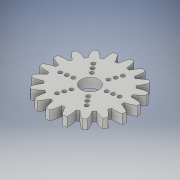
# Autodesk Inventor part: 000.303 - Шестерня привода
Saved by Autodesk Inventor 2019 (Build 230136000, 136)
## iProperties
Created: 2020-02-27
Part Number: 000.303 - Шестерня привода
Material: Типовые
Document SubType Name: Modeling
Designer: Петров Иван
Density: 1 g/cm^3
Appearance: По умолчанию
Author: Петров Иван
Autodesk Inventor part; units mm, degrees
ref_plane "YZ Plane" through (0, 0, 0) normal (1, 0, 0) x (0, 1, 0)
ref_plane "XZ Plane" through (0, 0, 0) normal (0, 1, 0) x (-1, 0, 0)
ref_plane "XY Plane" through (0, 0, 0) normal (0, 0, 1) x (1, 0, 0)
sketch "Эскиз1" plane through (0, 0, 0) normal (0, 1, 0) x (-1, 0, 0)
  arc A0 (-8.6049, 20.7741) -> (-8.0517, 15.4673) centre (8.9595, 19.9228) ccw
  arc A1 (-8.0517, 15.4673) -> (-9.3692, 14.7066) centre (0, 0) ccw
  arc A2 (-9.3692, 14.7066) -> (-13.6885, 17.8391) centre (-21.7334, 2.2022) ccw
  arc A3 (-13.6885, 17.8391) -> (-15.1912, 16.5782) centre (0, 0) ccw
  arc A4 (-15.1912, 16.5782) -> (-12.8563, 11.7806) centre (1.6052, 21.7856) ccw
  arc A5 (-12.8563, 11.7806) -> (-13.8341, 10.6153) centre (0, 0) ccw
  arc A6 (-13.8341, 10.6153) -> (-18.9643, 12.0816) centre (-21.1759, -5.3638) ccw
  arc A7 (-18.9643, 12.0816) -> (-19.9451, 10.3828) centre (0, 0) ccw
  arc A8 (-19.9451, 10.3828) -> (-16.1101, 6.673) centre (-5.9427, 21.0208) ccw
  arc A9 (-16.1101, 6.673) -> (-16.6304, 5.2436) centre (0, 0) ccw
  arc A10 (-16.6304, 5.2436) -> (-21.9528, 4.8668) centre (-18.0643, -12.2829) ccw
  arc A11 (-21.9528, 4.8668) -> (-22.2934, 2.935) centre (0, 0) ccw
  arc A12 (-22.2934, 2.935) -> (-17.4209, 0.7606) centre (-12.7739, 17.7205) ccw
  arc A13 (-17.4209, 0.7606) -> (-17.4209, -0.7606) centre (0, 0) ccw
  arc A14 (-17.4209, -0.7606) -> (-22.2934, -2.935) centre (-12.7739, -17.7205) ccw
  arc A15 (-22.2934, -2.935) -> (-21.9528, -4.8668) centre (0, 0) ccw
  arc A16 (-21.9528, -4.8668) -> (-16.6304, -5.2436) centre (-18.0643, 12.2829) ccw
  arc A17 (-16.6304, -5.2436) -> (-16.1101, -6.673) centre (0, 0) ccw
  arc A18 (-16.1101, -6.673) -> (-19.9451, -10.3828) centre (-5.9427, -21.0208) ccw
  arc A19 (-19.9451, -10.3828) -> (-18.9643, -12.0816) centre (0, 0) ccw
  arc A20 (-18.9643, -12.0816) -> (-13.8341, -10.6153) centre (-21.1759, 5.3638) ccw
  arc A21 (-13.8341, -10.6153) -> (-12.8563, -11.7806) centre (0, 0) ccw
  arc A22 (-12.8563, -11.7806) -> (-15.1912, -16.5782) centre (1.6052, -21.7856) ccw
  arc A23 (-15.1912, -16.5782) -> (-13.6885, -17.8391) centre (0, 0) ccw
  arc A24 (-13.6885, -17.8391) -> (-9.3692, -14.7066) centre (-21.7334, -2.2022) ccw
  arc A25 (-9.3692, -14.7066) -> (-8.0517, -15.4673) centre (0, 0) ccw
  arc A26 (-8.0517, -15.4673) -> (-8.6049, -20.7741) centre (8.9595, -19.9228) ccw
  arc A27 (-8.6049, -20.7741) -> (-6.7616, -21.445) centre (0, 0) ccw
  arc A28 (-6.7616, -21.445) -> (-3.7742, -17.0242) centre (-19.6695, -9.5027) ccw
  arc A29 (-3.7742, -17.0242) -> (-2.2761, -17.2883) centre (0, 0) ccw
  arc A30 (-2.2761, -17.2883) -> (-0.9808, -22.4644) centre (15.2332, -15.6569) ccw
  arc A31 (-0.9808, -22.4644) -> (0.9808, -22.4644) centre (0, 0) ccw
  arc A32 (0.9808, -22.4644) -> (2.2761, -17.2883) centre (-15.2332, -15.6569) ccw
  arc A33 (2.2761, -17.2883) -> (3.7742, -17.0242) centre (0, 0) ccw
  arc A34 (3.7742, -17.0242) -> (6.7616, -21.445) centre (19.6695, -9.5027) ccw
  arc A35 (6.7616, -21.445) -> (8.6049, -20.7741) centre (0, 0) ccw
  arc A36 (8.6049, -20.7741) -> (8.0517, -15.4673) centre (-8.9595, -19.9228) ccw
  arc A37 (8.0517, -15.4673) -> (9.3692, -14.7066) centre (0, 0) ccw
  arc A38 (9.3692, -14.7066) -> (13.6885, -17.8391) centre (21.7334, -2.2022) ccw
  arc A39 (13.6885, -17.8391) -> (15.1912, -16.5782) centre (0, 0) ccw
  arc A40 (15.1912, -16.5782) -> (12.8563, -11.7806) centre (-1.6052, -21.7856) ccw
  arc A41 (12.8563, -11.7806) -> (13.8341, -10.6153) centre (0, 0) ccw
  arc A42 (13.8341, -10.6153) -> (18.9643, -12.0816) centre (21.1759, 5.3638) ccw
  arc A43 (18.9643, -12.0816) -> (19.9451, -10.3828) centre (0, 0) ccw
  arc A44 (19.9451, -10.3828) -> (16.1101, -6.673) centre (5.9427, -21.0208) ccw
  arc A45 (16.1101, -6.673) -> (16.6304, -5.2436) centre (0, 0) ccw
  arc A46 (16.6304, -5.2436) -> (21.9528, -4.8668) centre (18.0643, 12.2829) ccw
  arc A47 (21.9528, -4.8668) -> (22.2934, -2.935) centre (0, 0) ccw
  arc A48 (22.2934, -2.935) -> (17.4209, -0.7606) centre (12.7739, -17.7205) ccw
  arc A49 (17.4209, -0.7606) -> (17.4209, 0.7606) centre (0, 0) ccw
  arc A50 (17.4209, 0.7606) -> (22.2934, 2.935) centre (12.7739, 17.7205) ccw
  arc A51 (22.2934, 2.935) -> (21.9528, 4.8668) centre (0, 0) ccw
  arc A52 (21.9528, 4.8668) -> (16.6304, 5.2436) centre (18.0643, -12.2829) ccw
  arc A53 (16.6304, 5.2436) -> (16.1101, 6.673) centre (0, 0) ccw
  arc A54 (16.1101, 6.673) -> (19.9451, 10.3828) centre (5.9427, 21.0208) ccw
  arc A55 (19.9451, 10.3828) -> (18.9643, 12.0816) centre (0, 0) ccw
  arc A56 (18.9643, 12.0816) -> (13.8341, 10.6153) centre (21.1759, -5.3638) ccw
  arc A57 (13.8341, 10.6153) -> (12.8563, 11.7806) centre (0, 0) ccw
  arc A58 (12.8563, 11.7806) -> (15.1912, 16.5782) centre (-1.6052, 21.7856) ccw
  arc A59 (15.1912, 16.5782) -> (13.6885, 17.8391) centre (0, 0) ccw
  arc A60 (13.6885, 17.8391) -> (9.3692, 14.7066) centre (21.7334, 2.2022) ccw
  arc A61 (9.3692, 14.7066) -> (8.0517, 15.4673) centre (0, 0) ccw
  arc A62 (8.0517, 15.4673) -> (8.6049, 20.7741) centre (-8.9595, 19.9228) ccw
  arc A63 (8.6049, 20.7741) -> (6.7616, 21.445) centre (0, 0) ccw
  arc A64 (6.7616, 21.445) -> (3.7742, 17.0242) centre (19.6695, 9.5027) ccw
  arc A65 (3.7742, 17.0242) -> (2.2761, 17.2883) centre (0, 0) ccw
  arc A66 (2.2761, 17.2883) -> (0.9808, 22.4644) centre (-15.2332, 15.6569) ccw
  arc A67 (0.9808, 22.4644) -> (-0.9808, 22.4644) centre (0, 0) ccw
  arc A68 (-0.9808, 22.4644) -> (-2.2761, 17.2883) centre (15.2332, 15.6569) ccw
  arc A69 (-2.2761, 17.2883) -> (-3.7742, 17.0242) centre (0, 0) ccw
  arc A70 (-3.7742, 17.0242) -> (-6.7616, 21.445) centre (-19.6695, 9.5027) ccw
  arc A71 (-6.7616, 21.445) -> (-8.6049, 20.7741) centre (0, 0) ccw
  constraints: 144 point on circle, 72 centre point
extrude "Выдавливание1" add sketch "Эскиз1" along normal blind 5
sketch "Эскиз2" plane through (0, 5, 0) normal (0, 1, 0) x (1, 0, 0)
  arc A0 (14.2029, 0.3107) -> (13.9664, 4.3996) centre (13.4768, 2.32) ccw
  line L0 (13.9664, 4.3996) -> (5.393, 4.3996)
  line L1 (5.393, 4.3996) -> (6.8323, 12.4554)
  arc A1 (6.8323, 12.4554) -> (3.173, 14.2951) centre (4.7292, 12.8312) ccw
  line L2 (3.173, 14.2951) -> (-1.1137, 6.8702)
  line L3 (-1.1137, 6.8702) -> (-7.3706, 12.1447)
  arc A2 (-7.3706, 12.1447) -> (-10.7934, 9.8955) centre (-8.7476, 10.5112) ccw
  line L4 (-10.7934, 9.8955) -> (-6.5067, 2.4706)
  line L5 (-6.5067, 2.4706) -> (-14.2029, -0.3107)
  arc A3 (-14.2029, -0.3107) -> (-13.9664, -4.3996) centre (-13.4768, -2.32) ccw
  line L6 (-13.9664, -4.3996) -> (-5.393, -4.3996)
  line L7 (-5.393, -4.3996) -> (-6.8323, -12.4554)
  arc A4 (-6.8323, -12.4554) -> (-3.173, -14.2951) centre (-4.7292, -12.8312) ccw
  line L8 (-3.173, -14.2951) -> (1.1137, -6.8702)
  line L9 (1.1137, -6.8702) -> (7.3706, -12.1447)
  arc A5 (7.3706, -12.1447) -> (10.7934, -9.8955) centre (8.7476, -10.5112) ccw
  line L10 (10.7934, -9.8955) -> (6.5067, -2.4706)
  line L11 (6.5067, -2.4706) -> (14.2029, 0.3107)
  circle A6 centre (7.5637, 1.3021) radius 1
  circle A7 centre (13.4768, 2.32) radius 1
  circle A8 centre (6.8286, -8.2053) radius 1
  circle A9 centre (-2.6542, -7.2014) radius 1
  circle A10 centre (-4.7292, -12.8312) radius 1
  circle A11 centre (-10.5203, -1.8111) radius 1
  circle A12 centre (-4.9095, 5.8993) radius 1
  circle A13 centre (-8.7476, 10.5112) radius 1
  circle A14 centre (3.6917, 10.0163) radius 1
  circle A15 centre (0, 0) radius 4.75
  circle A16 centre (4.7292, 12.8312) radius 1
  circle A17 centre (2.6542, 7.2014) radius 1
  circle A18 centre (-6.8286, 8.2053) radius 1
  circle A19 centre (-13.4768, -2.32) radius 1
  circle A20 centre (-7.5637, -1.3021) radius 1
  circle A21 centre (-3.6917, -10.0163) radius 1
  circle A22 centre (8.7476, -10.5112) radius 1
  circle A23 centre (4.9095, -5.8993) radius 1
  circle A24 centre (10.5203, 1.8111) radius 1
  circle A25 centre (0, 0) radius 1.875
  constraints: 26 centre point, 24 end point, 12 point on circle
extrude "Выдавливание2" cut sketch "Эскиз2" against normal blind 10 contours A6 | A7 | A8 | A9 | A10 | A11 | A12 | A13 | A14 | A15 | A16 | A17 | A18 | A19 | A20 | A21 | A22 | A23 | A24 | A25
